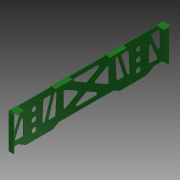
# Autodesk Inventor part: InnerSide 2
Saved by Autodesk Inventor 2015 (Build 190159000, 159)
## iProperties
Created: 2014-01-11
Part Number: InnerSide 2
Material: Generic
Document SubType Name: Sheet Metal
Designer: Alex
Density: 1 g/cm^3
Sheet Metal Rule: Default
Appearance: Smooth - Dark Forest Green
Mass: 262.954 g
Surface Area: 2370.16 cm^2
Volume: 262.954 cm^3
Author: Alex
Autodesk Inventor part; units mm, degrees
ref_plane "YZ Plane" through (0, 0, 0) normal (1, 0, 0) x (0, 1, 0)
ref_plane "XZ Plane" through (0, 0, 0) normal (0, 1, 0) x (-1, 0, 0)
ref_plane "XY Plane" through (0, 0, 0) normal (0, 0, 1) x (1, 0, 0)
sketch "Sketch1" plane through (0, 0, 0) normal (1, 0, 0) x (0, 1, 0)
  line L0 (196.2698, 454.4639) -> (43.8698, 454.4639)
  line L1 (43.8698, 454.4639) -> (43.8698, -237.9401)
  line L2 (43.8698, -237.9401) -> (196.2698, -237.9401)
  line L3 (196.2698, -237.9401) -> (196.2698, 454.4639)
  point P0 (0, 0)
  dimension "d0" = 152.4
  dimension "d1" = 692.404
  measures "d0" distance of L2.end L1.end
  measures "d1" distance of L1.end L0.end
extrude "Plate1" add sketch "Sketch1" along normal blind 2.286
sketch "Sketch2" plane through (0, 43.8698, 452.1779) normal (0, 0, 1) x (1, 0, 0)
  line L0 (0, 152.4) -> (0, 0)
  line L1 (0, 0) -> (25.4, 0)
  line L2 (25.4, 0) -> (25.4, 152.4)
  line L3 (25.4, 152.4) -> (0, 152.4)
  constraints: 6 end point, 1 horizontal, 1 perpendicular, 1 vertical
edge flange "Flange1" height 25.4 angle 90 thickness 2.286 bend radius 2.286 thickness toward (0, 0, 1) relief straight relief width 2.286 relief depth 1.143 corner gap 2.286 corner form 0 edges at (2.286, 120.0698, 454.4639) (2.286, 120.0698, -237.9401) wall of the first edge with corners at (0, 196.2698, 452.1779) (0, 43.8698, 452.1779) (25.4, 43.8698, 452.1779) (25.4, 196.2698, 452.1779)
bend "Bend1"
corner "Corner1"
sketch "Sketch3" plane through (0, 0, 0) normal (-1, 0, 0) x (0, 0, 1)
  line L0 (449.8919, 43.8698) -> (-233.3681, 43.8698) projected
  line L1 (-13.9121, 120.0698) -> (-13.9121, 196.2698) projected
  line L2 (-13.9121, 120.0698) -> (-11.6261, 120.0698) projected
  line L3 (-11.6261, 196.2698) -> (-11.6261, 120.0698) projected
  line L4 (-13.9121, 196.2698) -> (-11.6261, 196.2698) projected
  line L5 (228.1499, 120.0698) -> (228.1499, 196.2698) projected
  line L6 (228.1499, 120.0698) -> (230.4359, 120.0698) projected
  line L7 (230.4359, 196.2698) -> (230.4359, 120.0698) projected
  line L8 (228.1499, 196.2698) -> (230.4359, 196.2698) projected
  line L9 (-11.6261, 120.0698) -> (-13.9121, 120.0698)
  line L10 (-13.9121, 120.0698) -> (-13.9121, 43.8698)
  line L11 (-13.9121, 43.8698) -> (-11.6261, 43.8698)
  line L12 (-11.6261, 43.8698) -> (-11.6261, 120.0698)
  line L13 (230.4359, 120.0698) -> (228.1499, 120.0698)
  line L14 (228.1499, 120.0698) -> (228.1499, 43.8698)
  line L15 (228.1499, 43.8698) -> (230.4359, 43.8698)
  line L16 (230.4359, 43.8698) -> (230.4359, 120.0698)
  line L17 (-13.9121, 120.0698) -> (-11.6261, 120.0698)
  line L18 (-11.6261, 120.0698) -> (-11.6261, 43.8698)
  line L19 (-11.6261, 43.8698) -> (-13.9121, 43.8698)
  line L20 (-13.9121, 43.8698) -> (-13.9121, 120.0698)
  line L21 (228.1499, 120.0698) -> (230.4359, 120.0698)
  line L22 (230.4359, 120.0698) -> (230.4359, 43.8698)
  line L23 (230.4359, 43.8698) -> (228.1499, 43.8698)
  line L24 (228.1499, 43.8698) -> (228.1499, 120.0698)
  point P0 (0, 0)
  constraints: 32 end point, 8 parallel, 4 horizontal, 4 perpendicular, 2 point on line
extrude "Cut1" cut sketch "Sketch3" against normal blind 2.286 contours L0 L14 L6 L16 | L0 L10 L2 L12
sketch "Sketch7" plane through (0, 0, 0) normal (-1, 0, 0) x (0, 0, 1)
  line L0 (-233.3681, 196.2698) -> (449.8919, 196.2698)
  line L1 (-233.3681, 196.2698) -> (-202.1261, 196.2698)
  line L2 (-202.1261, 196.2698) -> (-202.1261, 198.5558)
  line L3 (-202.1261, 198.5558) -> (-233.3681, 198.5558)
  line L4 (-233.3681, 198.5558) -> (-233.3681, 196.2698)
  line L5 (449.8919, 196.2698) -> (418.6499, 196.2698)
  line L6 (418.6499, 196.2698) -> (418.6499, 198.5558)
  line L7 (418.6499, 198.5558) -> (449.8919, 198.5558)
  line L8 (449.8919, 198.5558) -> (449.8919, 196.2698)
  point P0 (-52.0121, 196.2698)
  point P1 (0, 0)
  dimension "d50" = 31.242
  dimension "d51" = 2.286
  dimension "d52" = 31.242
  dimension "d53" = 2.286
  measures "d50" distance of L3.end L2.end
  measures "d51" distance between parallel lines of L3 L0
  measures "d52" distance of L6.end L7.end
  measures "d53" distance between parallel lines of L5 L7
sheet face with bend "Face2" sketch "Sketch7" thickness 2.286 toward (1, 0, 0) bend radius 2.286 relief straight relief width 2.286 relief depth 1.143
bend "Bend3"
sketch "Sketch8" plane through (2.286, 198.5558, -202.1261) normal (0, 1, 0) x (-1, 0, 0)
  line L0 (0, -31.242) -> (0, 0)
  line L1 (0, 0) -> (-35.814, 0)
  line L2 (-35.814, 0) -> (-35.814, -31.242)
  line L3 (-35.814, -31.242) -> (0, -31.242)
  constraints: 6 end point, 1 horizontal, 1 perpendicular, 1 vertical
edge flange "Flange3" height 38.1 angle 90 thickness 2.286 bend radius 2.286 thickness toward (0, 1, 0) relief straight relief width 2.286 relief depth 1.143 corner gap 2.286 corner form 0 edges at (2.286, 198.5558, -217.7471) (2.286, 198.5558, 434.2709) wall of the first edge with corners at (2.286, 198.5558, -233.3681) (2.286, 198.5558, -202.1261) (38.1, 198.5558, -202.1261) (38.1, 198.5558, -233.3681)
bend "Bend4"
corner "Corner3"
sketch "Sketch9" plane through (0, 0, 0) normal (-1, 0, 0) x (0, 0, 1)
  line L0 (-50.8691, 196.2698) -> (25.3309, 196.2698)
  line L1 (25.3309, 196.2698) -> (25.3309, 198.5558)
  line L2 (25.3309, 198.5558) -> (-50.8691, 198.5558)
  line L3 (-50.8691, 198.5558) -> (-50.8691, 196.2698)
  line L4 (191.1929, 196.2698) -> (267.3929, 196.2698)
  line L5 (267.3929, 196.2698) -> (267.3929, 198.5558)
  line L6 (267.3929, 198.5558) -> (191.1929, 198.5558)
  line L7 (191.1929, 198.5558) -> (191.1929, 196.2698)
  point P0 (0, 0)
  point P1 (267.3929, 196.2698)
  point P2 (25.3309, 196.2698)
  dimension "d69" = 2.286
  dimension "d70" = 2.286
  measures "d69" distance of L1.end L0.end
  measures "d70" distance of L5.end L4.end
sheet face with bend "Face3" sketch "Sketch9" thickness 2.286 toward (1, 0, 0) bend radius 2.286 relief straight relief width 2.286 relief depth 1.143
bend "Bend5"
sketch "Sketch10" plane through (2.286, 198.5558, 25.3309) normal (0, 1, 0) x (-1, 0, 0)
  line L0 (0, -76.2) -> (0, 0)
  line L1 (0, 0) -> (-23.114, 0)
  line L2 (-23.114, 0) -> (-23.114, -76.2)
  line L3 (-23.114, -76.2) -> (0, -76.2)
  constraints: 6 end point, 1 horizontal, 1 perpendicular, 1 vertical
edge flange "Flange4" height 25.4 angle 90 thickness 2.286 bend radius 2.286 thickness toward (0, 1, 0) relief straight relief width 2.286 relief depth 1.143 corner gap 2.286 corner form 0 edges at (2.286, 198.5558, -12.7691) (2.286, 198.5558, 229.2929) wall of the first edge with corners at (2.286, 198.5558, -50.8691) (2.286, 198.5558, 25.3309) (25.4, 198.5558, 25.3309) (25.4, 198.5558, -50.8691)
bend "Bend6"
corner "Corner4"
sketch "Sketch14" plane through (25.4, 43.8698, -237.9401) normal (0, 0, -1) x (-1, 0, 0)
  circle A0 centre (10.414, 50.8) radius 1.5875
  point P0 (25.4, -43.8698)
  constraints: 1 centre point, 2 other
extrude "Cut7" cut sketch "Sketch14" against normal through all
sketch "Sketch15" plane through (0, 0, 0) normal (-1, 0, 0) x (0, 0, 1)
  line L0 (449.8919, 43.8698) -> (230.4359, 43.8698) projected
  line L1 (-13.9121, 43.8698) -> (-233.3681, 43.8698) projected
  line L2 (449.8919, 48.4418) -> (403.6639, 48.4418)
  line L3 (-233.3681, 48.4418) -> (-187.1401, 48.4418)
  line L4 (-233.3681, 48.4418) -> (-187.0131, 48.4418)
  line L5 (-187.0131, 48.4418) -> (-187.0131, 43.8698)
  line L6 (-187.0131, 43.8698) -> (-233.3681, 43.8698)
  line L7 (-233.3681, 43.8698) -> (-233.3681, 48.4418)
  line L8 (449.8919, 48.4418) -> (403.5369, 48.4418)
  line L9 (403.5369, 48.4418) -> (403.5369, 43.8698)
  line L10 (403.5369, 43.8698) -> (449.8919, 43.8698)
  line L11 (449.8919, 43.8698) -> (449.8919, 48.4418)
  line L12 (449.8919, 48.4418) -> (403.6639, 48.4418)
  line L13 (449.8919, 48.4418) -> (403.6639, 48.4418)
  line L14 (-187.1401, 48.4418) -> (-233.3681, 48.4418)
  line L15 (-187.1401, 48.4418) -> (-233.3681, 48.4418)
  line L16 (-187.1401, 48.4418) -> (-233.3681, 48.4418)
  line L17 (-187.1401, 48.4418) -> (-233.3681, 48.4418)
  line L18 (-187.1401, 48.4418) -> (-233.3681, 48.4418)
  line L19 (-187.1401, 48.4418) -> (-233.3681, 48.4418)
  line L20 (-187.1401, 48.4418) -> (-233.3681, 48.4418)
  line L21 (228.1499, 43.8698) -> (-11.6261, 43.8698) projected
  line L22 (228.1499, 43.8698) -> (228.1499, 120.0698) projected
  line L23 (228.1499, 120.0698) -> (230.4359, 120.0698) projected
  line L24 (230.4359, 120.0698) -> (230.4359, 43.8698) projected
  line L25 (449.8919, 43.8698) -> (230.4359, 43.8698) projected
  line L26 (449.8919, 43.8698) -> (449.8919, 196.2698) projected
  line L27 (418.6499, 196.2698) -> (449.8919, 196.2698) projected
  line L28 (267.3929, 196.2698) -> (418.6499, 196.2698) projected
  line L29 (191.1929, 196.2698) -> (267.3929, 196.2698) projected
  line L30 (25.3309, 196.2698) -> (191.1929, 196.2698) projected
  line L31 (-50.8691, 196.2698) -> (25.3309, 196.2698) projected
  line L32 (-202.1261, 196.2698) -> (-50.8691, 196.2698) projected
  line L33 (-233.3681, 196.2698) -> (-202.1261, 196.2698) projected
  line L34 (-233.3681, 196.2698) -> (-233.3681, 43.8698) projected
  line L35 (-13.9121, 43.8698) -> (-13.9121, 120.0698) projected
  line L36 (-13.9121, 120.0698) -> (-11.6261, 120.0698) projected
  line L37 (-11.6261, 120.0698) -> (-11.6261, 43.8698) projected
  line L38 (-187.1401, 48.4418) -> (-233.3681, 48.4418)
  line L39 (-187.1401, 48.4418) -> (-233.3681, 48.4418)
  line L40 (-233.3681, 48.4418) -> (-187.1401, 48.4418)
  line L41 (-233.3681, 48.4418) -> (-187.1401, 48.4418)
  line L42 (-233.3681, 48.4418) -> (-187.1401, 48.4418)
  line L43 (-187.0131, 43.8698) -> (-241.061, 43.8698)
  line L44 (-241.061, 43.8698) -> (-241.061, 48.4418)
  line L45 (-241.061, 48.4418) -> (-187.0131, 48.4418)
  line L46 (-187.0131, 48.4418) -> (-187.0131, 43.8698)
  line L47 (403.5369, 43.8698) -> (457.1836, 43.8698)
  line L48 (457.1836, 43.8698) -> (457.1836, 48.4418)
  line L49 (457.1836, 48.4418) -> (403.5369, 48.4418)
  line L50 (403.5369, 48.4418) -> (403.5369, 43.8698)
  line L51 (-13.9121, 43.8698) -> (-233.3681, 43.8698) projected
  point P0 (0, 0)
  dimension "d96" = 46.355
  dimension "d97" = 46.355
  constraints: 64 end point, 20 horizontal, 8 parallel, 4 perpendicular, 4 point on line, 4 other
  measures "d96" distance of L3.start L4.end
  measures "d97" distance of L10.end L9.end
extrude "Cut8" cut sketch "Sketch15" against normal blind 2.286 contours L0 L9 L8 L2 L11 | L1 L7 L3 L4 L5
sketch "Sketch16" plane through (0, 0, 0) normal (-1, 0, 0) x (0, 0, 1)
  circle A0 centre (-26.8661, 120.0698) radius 1.5878
  circle A1 centre (1.3279, 120.0698) radius 1.5875
  circle A2 centre (-26.8661, 120.0698) radius 1.5878
  circle A3 centre (1.0612, 181.2838) radius 1.7907
  circle A4 centre (215.1959, 185.1573) radius 1.5875
  circle A5 centre (243.1232, 181.2838) radius 1.7859
  circle A6 centre (1.0612, 170.6706) radius 1.7859
  circle A7 centre (243.1232, 181.2838) radius 1.7859
  line L0 (1.0612, 181.2838) -> (243.1232, 181.2838) construction
  point P0 (0, 0)
  point P1 (-12.7754, 170.6706)
  dimension "d104" = 3.5814
  constraints: 8 centre point, 2 end point, 1 coincident, 1 concentric, 1 horizontal, 9 other
  measures "d104" diameter of A3
extrude "Cut9" cut sketch "Sketch16" against normal blind 2.286 contours A3 | A5
sketch "Sketch18" plane through (2.286, 0, 0) normal (1, 0, 0) x (0, 0, -1)
  line L0 (-403.5369, 48.4418) -> (-403.5369, 43.8698)
  line L1 (-230.4359, 43.8698) -> (-230.4359, 120.0698)
  line L2 (-377.1405, 28.6298) -> (-256.8324, 28.6298)
  line L3 (-403.5369, 43.8698) -> (-230.4359, 43.8698)
  line L4 (-230.4359, 43.8698) -> (-256.8324, 28.6298)
  line L5 (-403.5369, 43.8698) -> (-377.1405, 28.6298)
  line L6 (13.9121, 120.0698) -> (13.9121, 43.8698)
  line L7 (187.0131, 43.8698) -> (13.9121, 43.8698)
  line L8 (187.0131, 43.8698) -> (187.0131, 48.4418)
  line L9 (40.3085, 28.6298) -> (160.6166, 28.6298)
  line L10 (13.9121, 43.8698) -> (40.3085, 28.6298)
  line L11 (160.6166, 28.6298) -> (187.0131, 43.8698)
  point P0 (0, 0)
  dimension "d121" = 15.24
  dimension "d127" = 30
  dimension "d128" = 30
  dimension "d129" = 15.24
  dimension "d130" = 30
  dimension "d131" = 30
  measures "d121" distance between parallel lines of L3 L2
  measures "d127" angle of L3 L5
  measures "d128" angle of L3 L4
  measures "d129" distance between parallel lines of L9 L7
  measures "d130" angle of L7 L10
  measures "d131" angle of L7 L11
sheet face with bend "Face4" sketch "Sketch18" thickness 2.286 toward (-1, 0, 0) bend radius 2.286 relief straight relief width 2.286 relief depth 1.143
bend "Bend7"
sketch "Sketch19" plane through (2.286, 0, 0) normal (1, 0, 0) x (0, 0, -1)
  circle A0 centre (91.9028, 165.1548) radius 2.5527
  circle A1 centre (98.2528, 148.6448) radius 2.5273
  circle A2 centre (123.6528, 148.6448) radius 10.414
  line L0 (85.5528, 169.9808) -> (85.5528, 33.3288)
  line L1 (85.5528, 33.3288) -> (87.0768, 31.8048)
  line L2 (160.2288, 31.8048) -> (87.0768, 31.8048)
  line L3 (160.2288, 31.8048) -> (161.7528, 33.3288)
  line L4 (161.7528, 169.9808) -> (161.7528, 33.3288)
  line L5 (161.7528, 169.9808) -> (160.2288, 171.5048)
  line L6 (160.2288, 171.5048) -> (87.0768, 171.5048)
  line L7 (87.0768, 171.5048) -> (85.5528, 169.9808)
  circle A3 centre (149.0528, 148.6448) radius 2.5273
  circle A4 centre (155.4028, 165.1548) radius 2.5527
  circle A5 centre (91.9028, 38.1548) radius 2.5527
  circle A6 centre (104.6028, 62.4372) radius 1.9837
  circle A7 centre (142.7028, 62.4372) radius 1.9837
  circle A8 centre (155.4028, 38.1548) radius 2.5527
  circle A9 centre (123.6528, 107.9286) radius 11.1061
  line L8 (160.6166, 28.6298) -> (40.3085, 28.6298) projected
  line L9 (13.9121, 120.0698) -> (13.9121, 43.8698) projected
  circle A10 centre (-371.9139, 165.1548) radius 2.5527
  circle A11 centre (-365.5639, 148.6448) radius 2.5273
  circle A12 centre (-340.1639, 148.6448) radius 10.414
  circle A13 centre (-340.1639, 107.9286) radius 11.1061
  line L10 (-378.2639, 169.9808) -> (-378.2639, 33.3288)
  line L11 (-302.0639, 169.9808) -> (-302.0639, 33.3288)
  circle A14 centre (-321.1139, 62.4372) radius 1.9837
  circle A15 centre (-359.2139, 62.4372) radius 1.9837
  circle A16 centre (-308.4139, 38.1548) radius 2.5527
  line L12 (-303.5879, 31.8048) -> (-302.0639, 33.3288)
  circle A17 centre (-371.9139, 38.1548) radius 2.5527
  line L13 (-303.5879, 31.8048) -> (-376.7399, 31.8048)
  line L14 (-378.2639, 33.3288) -> (-376.7399, 31.8048)
  circle A18 centre (-314.7639, 148.6448) radius 2.5273
  line L15 (-376.7399, 171.5048) -> (-378.2639, 169.9808)
  line L16 (-303.5879, 171.5048) -> (-376.7399, 171.5048)
  line L17 (-302.0639, 169.9808) -> (-303.5879, 171.5048)
  circle A19 centre (-308.4139, 165.1548) radius 2.5527
  line L18 (-403.5369, 48.4418) -> (-403.5369, 43.8698) projected
  line L19 (-256.8324, 28.6298) -> (-377.1405, 28.6298) projected
  circle A20 centre (-340.1639, 67.2128) radius 11.1125
  circle A21 centre (123.6528, 67.2128) radius 11.1125
  point P0 (0, 0)
  point P1 (1.5875, 1.5875)
  dimension "d135" = 20.828
  dimension "d136" = 22.2123
  dimension "d146" = 5.1054
  dimension "d147" = 5.1054
  dimension "d148" = 5.0546
  dimension "d149" = 5.0546
  dimension "d150" = 3.9675
  dimension "d151" = 3.9675
  dimension "d152" = 5.1054
  dimension "d153" = 5.1054
  dimension "d154" = 73.152
  dimension "d155" = 136.652
  dimension "d156" = 136.652
  dimension "d157" = 73.152
  dimension "d158" = 1.524
  dimension "d159" = 1.524
  dimension "d160" = 1.524
  dimension "d161" = 1.524
  dimension "d162" = 1.524
  dimension "d163" = 1.524
  dimension "d164" = 1.524
  dimension "d165" = 1.524
  dimension "d166" = 6.35
  dimension "d167" = 6.35
  dimension "d168" = 6.35
  dimension "d169" = 6.35
  dimension "d170" = 30.6324
  dimension "d171" = 19.05
  dimension "d172" = 19.05
  dimension "d173" = 30.6324
  dimension "d174" = 38.1
  dimension "d175" = 63.5762
  dimension "d176" = 38.1
  dimension "d177" = 22.86
  dimension "d178" = 12.7
  dimension "d179" = 22.86
  dimension "d180" = 6.35
  dimension "d181" = 6.35
  dimension "d182" = 6.35
  dimension "d183" = 6.35
  dimension "d184" = 12.7
  dimension "d185" = 22.86
  dimension "d186" = 3.175
  dimension "d187" = 71.6407
  dimension "d188" = 20.828
  dimension "d189" = 22.2123
  dimension "d191" = 5.1054
  dimension "d192" = 5.1054
  dimension "d193" = 5.0546
  dimension "d194" = 5.0546
  dimension "d195" = 3.9675
  dimension "d196" = 3.9675
  dimension "d197" = 5.1054
  dimension "d198" = 5.1054
  dimension "d199" = 73.152
  dimension "d200" = 136.652
  dimension "d201" = 136.652
  dimension "d202" = 73.152
  dimension "d203" = 1.524
  dimension "d204" = 1.524
  dimension "d205" = 1.524
  dimension "d206" = 1.524
  dimension "d207" = 1.524
  dimension "d208" = 1.524
  constraints: 32 end point, 22 centre point, 4 parallel
  measures "d135" diameter of A2
  measures "d136" diameter of A9
  measures "d146" diameter of A0
  measures "d147" diameter of A4
  measures "d148" diameter of A3
  measures "d149" diameter of A1
  measures "d150" diameter of A6
  measures "d151" diameter of A7
  measures "d152" diameter of A5
  measures "d153" diameter of A8
  measures "d154" distance of L6.start L7.start
  measures "d155" distance of L4.start L4.end
  measures "d156" distance of L0.start L0.end
  measures "d157" distance of L3.start L2.end
  measures "d158" horizontal distance of L0.end L2.end
  measures "d159" horizontal distance of L0.end L2.end
  measures "d160" horizontal distance of L3.start L4.end
  measures "d161" horizontal distance of L3.start L4.end
  measures "d162" horizontal distance of L4.start L6.start
  measures "d163" horizontal distance of L4.start L6.start
  measures "d164" horizontal distance of L7.start L0.start
  measures "d165" horizontal distance of L7.start L0.start
  measures "d166" distance from line of L2 A5.centre
  measures "d167" distance from line of L0 A5.centre
  measures "d168" distance from line of L2 A8.centre
  measures "d169" distance from line of L4 A8.centre
  measures "d170" distance from line of L2 A6.centre
  measures "d171" distance from line of L0 A6.centre
  measures "d172" distance from line of L4 A7.centre
  measures "d173" distance from line of L2 A7.centre
  measures "d174" distance from line of L4 A9.centre
  measures "d175" distance from line of L6 A9.centre
  measures "d176" distance from line of L4 A2.centre
  measures "d177" distance from line of L6 A2.centre
  measures "d178" distance from line of L4 A3.centre
  measures "d179" distance from line of L6 A3.centre
  measures "d180" distance from line of L4 A4.centre
  measures "d181" distance from line of L6 A4.centre
  measures "d182" distance from line of L6 A0.centre
  measures "d183" distance from line of L0 A0.centre
  measures "d184" distance from line of L0 A1.centre
  measures "d185" distance from line of L6 A1.centre
  measures "d186" distance from line of L8 L2.end
  measures "d187" distance from line of L9 L0.end
  measures "d188" diameter of A12
  measures "d189" diameter of A13
  measures "d191" diameter of A10
  measures "d192" diameter of A19
  measures "d193" diameter of A18
  measures "d194" diameter of A11
  measures "d195" diameter of A15
  measures "d196" diameter of A14
  measures "d197" diameter of A17
  measures "d198" diameter of A16
  measures "d199" distance of L16.start L16.end
  measures "d200" distance of L11.start L12.end
  measures "d201" distance of L10.start L10.end
  measures "d202" distance of L13.start L13.end
  measures "d203" horizontal distance of L10.end L13.end
  measures "d204" horizontal distance of L10.end L13.end
  measures "d205" horizontal distance of L13.start L12.end
  measures "d206" horizontal distance of L13.start L12.end
  measures "d207" horizontal distance of L11.start L16.start
  measures "d208" horizontal distance of L11.start L16.start
extrude "Cut10" cut sketch "Sketch19" against normal blind 2.286 contours A0 | A1 | A2 | A3 | A4 | A5 | A6 | A7 | A8 | A9 | A10 | A11 | A12 | A13 | A14 | A15 | A16 | A17 | A18 | A19 | A20 | A21
sketch "Sketch21" plane through (0, 0, 0) normal (-1, 0, 0) x (0, 0, 1)
  line L0 (7.4239, 62.9198) -> (7.4239, 145.0823) projected
  line L1 (7.4239, 155.9801) -> (171.6236, 62.9198) projected
  arc A0 (16.9049, 150.6067) -> (7.4239, 145.0823) centre (13.7739, 145.0823) ccw projected
  arc A1 (66.6925, 111.3407) -> (66.6925, 122.3896) centre (63.5615, 116.8651) ccw projected
  arc A2 (7.4239, 88.6479) -> (16.9049, 83.1235) centre (13.7739, 88.6479) ccw projected
  line L2 (66.6925, 111.3407) -> (16.9049, 83.1235) projected
  line L3 (161.9807, 165.3453) -> (111.1877, 136.5584) projected
  arc A3 (104.9258, 136.5584) -> (111.1877, 136.5584) centre (108.0568, 142.0828) ccw projected
  line L4 (104.9258, 136.5584) -> (54.1328, 165.3453) projected
  arc A4 (57.2638, 177.2198) -> (54.1328, 165.3453) centre (57.2638, 170.8698) ccw projected
  line L5 (57.2638, 177.2198) -> (158.8497, 177.2198) projected
  arc A5 (161.9807, 165.3453) -> (158.8497, 177.2198) centre (158.8497, 170.8698) ccw projected
  line L6 (147.7644, 123.3284) -> (199.6189, 152.717) projected
  arc A6 (147.7644, 123.3284) -> (147.7644, 112.2795) centre (150.8954, 117.804) ccw projected
  line L7 (147.7644, 112.2795) -> (199.6189, 82.891) projected
  circle A7 centre (340.1639, 107.9286) radius 11.1061 projected
  circle A8 centre (308.4139, 165.1548) radius 2.5527 projected
  circle A9 centre (308.4139, 38.1548) radius 2.5527 projected
  circle A10 centre (365.5639, 148.6448) radius 2.5273 projected
  circle A11 centre (321.1139, 62.4372) radius 1.9837 projected
  circle A12 centre (-123.6528, 67.2128) radius 11.1125 projected
  circle A13 centre (-123.6528, 148.6448) radius 10.414 projected
  circle A14 centre (-91.9028, 38.1548) radius 2.5527 projected
  circle A15 centre (-91.9028, 165.1548) radius 2.5527 projected
  circle A16 centre (-98.2528, 148.6448) radius 2.5273 projected
  circle A17 centre (-142.7028, 62.4372) radius 1.9837 projected
  circle A18 centre (-104.6028, 62.4372) radius 1.9837 projected
  circle A19 centre (-149.0528, 148.6448) radius 2.5273 projected
  circle A20 centre (-155.4028, 38.1548) radius 2.5527 projected
  circle A21 centre (-155.4028, 165.1548) radius 2.5527 projected
  circle A22 centre (-123.6528, 107.9286) radius 11.1061 projected
  circle A23 centre (359.2139, 62.4372) radius 1.9837 projected
  circle A24 centre (314.7639, 148.6448) radius 2.5273 projected
  circle A25 centre (371.9139, 38.1548) radius 2.5527 projected
  circle A26 centre (371.9139, 165.1548) radius 2.5527 projected
  circle A27 centre (340.1639, 148.6448) radius 10.414 projected
  circle A28 centre (340.1639, 67.2128) radius 11.1125 projected
  circle A29 centre (243.1232, 181.2838) radius 1.7859 projected
  circle A30 centre (1.0612, 181.2838) radius 1.7907 projected
  line L8 (403.5369, 48.4418) -> (449.8919, 48.4418) projected
  line L9 (449.8919, 48.4418) -> (449.8919, 196.2698) projected
  line L10 (418.6499, 196.2698) -> (449.8919, 196.2698) projected
  line L11 (267.3929, 196.2698) -> (418.6499, 196.2698) projected
  line L12 (191.1929, 196.2698) -> (267.3929, 196.2698) projected
  line L13 (25.3309, 196.2698) -> (191.1929, 196.2698) projected
  line L14 (-50.8691, 196.2698) -> (25.3309, 196.2698) projected
  line L15 (-202.1261, 196.2698) -> (-50.8691, 196.2698) projected
  line L16 (-233.3681, 196.2698) -> (-202.1261, 196.2698) projected
  line L17 (-233.3681, 196.2698) -> (-233.3681, 48.4418) projected
  line L18 (-233.3681, 48.4418) -> (-187.0131, 48.4418) projected
  line L19 (-187.0131, 48.4418) -> (-187.0131, 43.8698) projected
  line L20 (-160.6166, 28.6298) -> (-187.0131, 43.8698) projected
  line L21 (-40.3085, 28.6298) -> (-160.6166, 28.6298) projected
  line L22 (-13.9121, 43.8698) -> (-40.3085, 28.6298) projected
  line L23 (-13.9121, 43.8698) -> (-13.9121, 120.0698) projected
  line L24 (-13.9121, 120.0698) -> (-11.6261, 120.0698) projected
  line L25 (-11.6261, 120.0698) -> (-11.6261, 43.8698) projected
  line L26 (228.1499, 43.8698) -> (-11.6261, 43.8698) projected
  line L27 (228.1499, 43.8698) -> (228.1499, 120.0698) projected
  line L28 (228.1499, 120.0698) -> (230.4359, 120.0698) projected
  line L29 (230.4359, 120.0698) -> (230.4359, 43.8698) projected
  line L30 (256.8324, 28.6298) -> (230.4359, 43.8698) projected
  line L31 (377.1405, 28.6298) -> (256.8324, 28.6298) projected
  line L32 (403.5369, 43.8698) -> (377.1405, 28.6298) projected
  line L33 (403.5369, 43.8698) -> (403.5369, 48.4418) projected
  line L34 (209.0999, 147.1926) -> (209.0999, 88.4154) projected
  arc A31 (199.6189, 82.891) -> (209.0999, 88.4154) centre (202.7499, 88.4154) ccw projected
  arc A32 (209.0999, 147.1926) -> (199.6189, 152.717) centre (202.7499, 147.1926) ccw projected
  arc A33 (147.5409, 62.9198) -> (150.6719, 74.7942) centre (147.5409, 69.2698) ccw projected
  line L35 (62.1285, 74.7942) -> (106.4002, 99.8852) projected
  arc A34 (109.5312, 98.1107) -> (103.2692, 98.1107) centre (106.4002, 92.5863) ccw projected
  arc A35 (62.1285, 74.7942) -> (65.2595, 62.9198) centre (65.2595, 69.2698) ccw projected
  line L36 (147.5409, 62.9198) -> (65.2595, 62.9198) projected
  point P0 (0, 0)
  point P1 (108.0568, 134.7839)
extrude "Cut13" cut sketch "Sketch21" against normal blind 2.286 contours L0 A0 L1 A1 L2 A2 | L1 A33 L36 A35 L35 A34 | L3 A3 L4 A4 L5 A5 | L6 A32 L34 A31 L7 A6
sketch "Sketch22" plane through (0, 0, 0) normal (-1, 0, 0) x (0, 0, 1)
  line L0 (-220.6681, 170.8698) -> (-220.6681, 111.0878)
  line L1 (-208.4828, 108.5834) -> (-182.8253, 168.3654)
  line L2 (-188.6606, 177.2198) -> (-214.3181, 177.2198)
  line L3 (-170.6555, 73.8418) -> (-170.6555, 133.6237)
  line L4 (-182.8408, 136.1281) -> (-208.4983, 76.3462)
  line L5 (-202.663, 67.4918) -> (-177.0055, 67.4918)
  line L6 (-202.1261, 196.2698) -> (-50.8691, 196.2698) projected
  line L7 (-233.3681, 196.2698) -> (-233.3681, 48.4418) projected
  line L8 (-233.3681, 48.4418) -> (-187.0131, 48.4418) projected
  line L9 (-157.9555, 127.2737) -> (-157.9555, 67.4918) construction
  circle A0 centre (-155.4028, 165.1548) radius 2.5527 projected
  circle A1 centre (-155.4028, 38.1548) radius 2.5527 construction
  line L10 (-40.3085, 28.6298) -> (-160.6166, 28.6298) construction
  arc A2 (-214.3181, 177.2198) -> (-220.6681, 170.8698) centre (-214.3181, 170.8698) ccw
  arc A3 (-220.6681, 111.0878) -> (-208.4828, 108.5834) centre (-214.3181, 111.0878) ccw
  arc A4 (-182.8253, 168.3654) -> (-188.6606, 177.2198) centre (-188.6606, 170.8698) ccw
  arc A5 (-170.6555, 133.6237) -> (-182.8408, 136.1281) centre (-177.0055, 133.6237) ccw
  arc A6 (-208.4983, 76.3462) -> (-202.663, 67.4918) centre (-202.663, 73.8418) ccw
  arc A7 (-177.0055, 67.4918) -> (-170.6555, 73.8418) centre (-177.0055, 73.8418) ccw
  line L11 (25.3309, 196.2698) -> (191.1929, 196.2698) projected
  line L12 (108.2619, 196.2698) -> (108.2619, 48.4418) construction
  line L13 (437.1919, 170.8698) -> (437.1919, 111.0878)
  line L14 (425.0066, 108.5834) -> (399.3491, 168.3654)
  line L15 (405.1844, 177.2198) -> (430.8419, 177.2198)
  line L16 (387.1793, 73.8418) -> (387.1793, 133.6237)
  line L17 (399.3646, 136.1281) -> (425.0221, 76.3462)
  line L18 (419.1868, 67.4918) -> (393.5293, 67.4918)
  line L19 (418.6499, 196.2698) -> (267.3929, 196.2698)
  line L20 (449.8919, 196.2698) -> (449.8919, 48.4418)
  line L21 (449.8919, 48.4418) -> (403.5369, 48.4418)
  line L22 (374.4793, 127.2737) -> (374.4793, 67.4918) construction
  circle A8 centre (371.9266, 165.1548) radius 2.5527
  circle A9 centre (371.9266, 38.1548) radius 2.5527 construction
  line L23 (256.8324, 28.6298) -> (377.1405, 28.6298) construction
  arc A10 (437.1919, 170.8698) -> (430.8419, 177.2198) centre (430.8419, 170.8698) ccw
  arc A11 (425.0066, 108.5834) -> (437.1919, 111.0878) centre (430.8419, 111.0878) ccw
  arc A12 (405.1844, 177.2198) -> (399.3491, 168.3654) centre (405.1844, 170.8698) ccw
  arc A13 (399.3646, 136.1281) -> (387.1793, 133.6237) centre (393.5293, 133.6237) ccw
  arc A14 (419.1868, 67.4918) -> (425.0221, 76.3462) centre (419.1868, 73.8418) ccw
  arc A15 (387.1793, 73.8418) -> (393.5293, 67.4918) centre (393.5293, 73.8418) ccw
  line L24 (299.6015, 160.5041) -> (303.011, 79.5034)
  line L25 (268.0313, 166.7978) -> (293.2291, 166.7978)
  arc A16 (273.3734, 73.1534) -> (276.1594, 81.1031) centre (270.2817, 78.6999) ccw
  arc A17 (290.5199, 77.7231) -> (303.011, 79.5034) centre (296.6385, 79.5034) ccw
  arc A18 (299.6015, 160.5041) -> (293.2291, 166.7978) centre (293.2517, 160.4479) ccw
  line L26 (290.5199, 77.7231) -> (265.1906, 158.828)
  line L27 (243.454, 77.6275) -> (238.5145, 161.7438)
  line L28 (250.8507, 162.1419) -> (276.1594, 81.1031)
  line L29 (273.3734, 73.1534) -> (248.0769, 73.1534)
  arc A19 (243.454, 77.6275) -> (248.0769, 73.1534) centre (249.573, 79.3247) ccw
  arc A20 (250.8507, 162.1419) -> (238.5145, 161.7438) centre (244.7308, 160.4478) ccw
  arc A21 (268.0313, 166.7978) -> (265.1906, 158.828) centre (271.0716, 161.223) ccw
  line L30 (229.455, 179.4978) -> (304.4094, 179.4978) construction
  circle A22 centre (243.1232, 181.2838) radius 1.7859 projected
  line L31 (334.3911, 60.4534) -> (287.3938, 60.4534) construction
  circle A23 centre (321.1139, 62.4372) radius 1.9837 projected
  line L32 (-51.5074, 166.7978) -> (-76.7053, 166.7978)
  arc A24 (-31.5531, 73.1534) -> (-26.9302, 77.6275) centre (-33.0492, 79.3247) ccw
  arc A25 (-59.6355, 81.1031) -> (-56.8496, 73.1534) centre (-53.7579, 78.6999) ccw
  line L33 (-56.8496, 73.1534) -> (-31.5531, 73.1534)
  arc A26 (-48.6667, 158.828) -> (-51.5074, 166.7978) centre (-54.5478, 161.223) ccw
  arc A27 (-76.7053, 166.7978) -> (-83.0777, 160.5041) centre (-76.7279, 160.4479) ccw
  arc A28 (-21.9907, 161.7438) -> (-34.3269, 162.1419) centre (-28.207, 160.4478) ccw
  line L34 (-73.9961, 77.7231) -> (-48.6667, 158.828)
  line L35 (-83.0777, 160.5041) -> (-86.4871, 79.5034)
  arc A29 (-86.4871, 79.5034) -> (-73.9961, 77.7231) centre (-80.1147, 79.5034) ccw
  line L36 (-26.9302, 77.6275) -> (-21.9907, 161.7438)
  line L37 (-34.3269, 162.1419) -> (-59.6355, 81.1031)
  line L38 (-12.9312, 179.4978) -> (-87.8855, 179.4978) construction
  circle A30 centre (-26.5994, 181.2838) radius 1.7859
  line L39 (-117.8673, 60.4534) -> (-70.87, 60.4534) construction
  circle A31 centre (-104.5901, 62.4372) radius 1.9837
  point P0 (0, 0)
  point P1 (-179.0251, 177.2198)
  point P2 (-170.6555, 164.5198)
  point P3 (395.5489, 177.2198)
  point P4 (387.1793, 164.5198)
  point P5 (262.7015, 166.7978)
  point P6 (235.6289, 210.8821)
  point P7 (-46.1777, 166.7978)
  dimension "d262" = 12.7
  dimension "d263" = 12.7
  dimension "d264" = 19.05
  dimension "d265" = 12.7
  dimension "d266" = 19.05
  dimension "d267" = 12.7
  dimension "d269" = 38.862
  dimension "d279" = 6.35
  dimension "d287" = 82.931
  dimension "d290" = 12.7
  dimension "d291" = 6.35
  dimension "d292" = 6.35
  dimension "d293" = 6.35
  dimension "d294" = 19.05
  dimension "d295" = 19.05
  dimension "d296" = 6.35
  dimension "d297" = 6.35
  dimension "d298" = 6.3724
  dimension "d299" = 12.7
  dimension "d300" = 12.7
  constraints: 70 end point, 56 symmetric about line, 48 point on circle, 28 centre point, 16 tangent, 14 point on line, 5 equal radius, 3 horizontal, 3 parallel, 2 vertical, 1 midpoint, 16 other
  measures "d262" distance between parallel lines of L4 L1
  measures "d263" vertical distance of point (-170.655, 164.52) point (-179.025, 177.22)
  measures "d264" distance between parallel lines of L6 L2
  measures "d265" distance between parallel lines of L7 L0
  measures "d266" distance between parallel lines of L8 L5
  measures "d267" distance between parallel lines of L9 L3
  measures "d269" distance from line of L10 L9.end
  measures "d279" radius of A2
  measures "d287" distance of L11.start L12.start
  measures "d290" distance between parallel lines of L29 L31
  measures "d291" radius of A16
  measures "d292" radius of A19
  measures "d293" radius of A20
  measures "d294" distance from line of A20.centre L30
  measures "d295" distance from line of A17.centre L31
  measures "d296" radius of A21
  measures "d297" radius of A18
  measures "d298" radius of A17
  measures "d299" distance between parallel lines of L30 L25
  measures "d300" distance between parallel lines of L37 L34
extrude "Cut14" cut sketch "Sketch22" against normal blind 2.286 contours A2 L2 A4 L1 A3 L0 | A7 L5 A6 L4 A5 L3 | L13 A11 L14 A12 L15 A10 | L16 A13 L17 A14 L18 A15 | L24 A17 L26 A21 L25 A18 | L29 A19 L27 A20 L28 A16 | A26 L34 A29 L35 A27 L32 | L33 A25 L37 A28 L36 A24
equation "\"d13\" = Thickness"
equation "\"d94\" = Thickness"
equation "\"d98\" = Thickness"
equation "\"d100\" = Thickness"
equation "\"TransitionRadius\" = BendRadius"
equation "\"d3\" = BendReliefWidth"
equation "\"d4\" = BendReliefDepth"
equation "\"d5\" = MinimumRemnant"
equation "\"d6\" = BendRadius"
equation "\"d9\" = BendRadius"
equation "\"d10\" = CornerReliefSize"
equation "\"d11\" = GapSize"
equation "\"d12\" = JacobiRadiusSize"
equation "\"d54\" = BendRadius"
equation "\"d55\" = BendReliefWidth"
equation "\"d57\" = MinimumRemnant"
equation "\"d56\" = BendReliefDepth"
equation "\"d58\" = BendRadius"
equation "\"d59\" = BendReliefWidth"
equation "\"d60\" = BendReliefDepth"
equation "\"d61\" = MinimumRemnant"
equation "\"d62\" = BendRadius"
equation "\"d65\" = BendRadius"
equation "\"d66\" = CornerReliefSize"
equation "\"d67\" = GapSize"
equation "\"d68\" = JacobiRadiusSize"
equation "\"d71\" = BendRadius"
equation "\"d72\" = BendReliefWidth"
equation "\"d74\" = MinimumRemnant"
equation "\"d73\" = BendReliefDepth"
equation "\"d75\" = BendRadius"
equation "\"d76\" = BendReliefWidth"
equation "\"d77\" = BendReliefDepth"
equation "\"d78\" = MinimumRemnant"
equation "\"d79\" = BendRadius"
equation "\"d82\" = BendRadius"
equation "\"d83\" = CornerReliefSize"
equation "\"d84\" = GapSize"
equation "\"d85\" = JacobiRadiusSize"
equation "\"BendRadius\" = Thickness"
equation "\"BendReliefWidth\" = Thickness"
equation "\"BendReliefDepth\" = 0.5 * Thickness"
equation "\"CornerReliefSize\" = 4 * Thickness"
equation "\"MinimumRemnant\" = 2 * Thickness"
equation "\"JacobiRadiusSize\" = BendRadius"
equation "\"GapSize\" = Thickness"
equation "\"d2\" = BendRadius"
equation "\"Thickness\" = 2.286"
body "Solid1"
